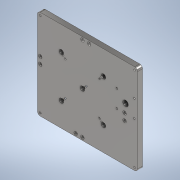
# Autodesk Inventor part: BasePlate
Saved by Autodesk Inventor 2022 (Build 260153070, 153G)
## iProperties
Company: UNC - Chapel Hill
Created: 2020-03-15
Part Number: BasePlate
Material: Stainless Steel
Document SubType Name: Modeling
Designer: elmar
Density: 8 g/cm^3
Appearance: Semi-Polished
BasePlateCornerRadius: 5.000 mm
BasePlateWidth: 160.000 mm
M3HoleDiameter: 3.200 mm
M3CounterSinkDiameter: 6.300 mm
MountHoleToSideDistance: 5.000 mm
Author: Eric L. Martin
Title: BasePlate
Autodesk Inventor part; units mm, degrees
ref_plane "YZ Plane" through (0, 0, 0) normal (1, 0, 0) x (0, 1, 0)
ref_plane "XZ Plane" through (0, 0, 0) normal (0, 1, 0) x (-1, 0, 0)
ref_plane "XY Plane" through (0, 0, 0) normal (0, 0, 1) x (1, 0, 0)
sketch "Sketch1" plane through (0, 0, 0) normal (0, 0, 1) x (1, 0, 0)
  line L0 (37.5, -37.5) -> (-37.5, -37.5)
  line L1 (-37.5, -37.5) -> (-37.5, 37.5)
  line L2 (-37.5, 37.5) -> (37.5, 37.5)
  line L3 (37.5, 37.5) -> (37.5, -37.5)
  line L4 (37.5, -37.5) -> (-37.5, 37.5) construction
  line L5 (-37.5, -37.5) -> (37.5, 37.5) construction
  line L6 (-75, 0) -> (0, 75)
  line L7 (0, 75) -> (75, 0)
  line L8 (75, 0) -> (0, -75)
  line L9 (0, -75) -> (-75, 0)
  line L10 (-115.5865, 0) -> (133.519, 0) projected
  circle A0 centre (37.5, 37.5) radius 37.5
  circle A1 centre (76.7825, 15.5482) radius 7.5
  circle A2 centre (37.5, -37.5) radius 38.5
  circle A3 centre (76.7825, 15.5482) radius 9.5
  line L11 (61.2825, 31.0482) -> (92.2825, 31.0482)
  line L12 (92.2825, 31.0482) -> (92.2825, 0.0482)
  line L13 (92.2825, 0.0482) -> (61.2825, 0.0482)
  line L14 (61.2825, 0.0482) -> (61.2825, 31.0482)
  line L15 (97.9325, 36.6982) -> (97.9325, -5.6018)
  line L16 (55.6325, -5.6018) -> (55.6325, 36.6982)
  line L17 (55.6325, 36.6982) -> (97.9325, 36.6982)
  line L18 (-80, 80) -> (97.9325, 80)
  line L19 (97.9325, 80) -> (97.9325, -80)
  line L20 (97.9325, -80) -> (-80, -80)
  line L21 (-80, -80) -> (-80, 80)
  circle A4 centre (76.7825, 15.5482) radius 11.5
  circle A5 centre (75, 0) radius 4.15
  circle A6 centre (61.2825, 0.0482) radius 4.15
  circle A7 centre (37.5, 37.5) radius 4
  circle A8 centre (0, 0) radius 4
  line L22 (3.9921, 0.2505) -> (0.2505, 3.9921)
  line L23 (37.2495, 33.5079) -> (33.5079, 37.2495)
  arc A9 (0.2505, 3.9921) -> (-1.3298, 3.7725) centre (-0.4566, 3.285) ccw
  arc A10 (3.7725, -1.3298) -> (3.9921, 0.2505) centre (3.285, -0.4566) ccw
  arc A11 (37.2495, 33.5079) -> (38.8298, 33.7275) centre (37.9566, 34.215) ccw
  arc A12 (33.7275, 38.8298) -> (33.5079, 37.2495) centre (34.215, 37.9566) ccw
  line L24 (36.7929, 34.6716) -> (34.6716, 32.5503)
  line L25 (34.6716, 32.5503) -> (32.5503, 34.6716)
  line L26 (32.5503, 34.6716) -> (34.6716, 36.7929)
  line L27 (34.6716, 36.7929) -> (36.7929, 34.6716)
  line L28 (36.7929, 34.6716) -> (32.5503, 34.6716) construction
  line L29 (34.6716, 32.5503) -> (34.6716, 36.7929) construction
  line L30 (2.8284, 0.7071) -> (4.9497, 2.8284)
  line L31 (4.9497, 2.8284) -> (2.8284, 4.9497)
  line L32 (2.8284, 4.9497) -> (0.7071, 2.8284)
  line L33 (0.7071, 2.8284) -> (2.8284, 0.7071)
  line L34 (2.8284, 0.7071) -> (2.8284, 4.9497) construction
  line L35 (4.9497, 2.8284) -> (0.7071, 2.8284) construction
  point P0 (-80, 0)
  point P1 (33.5, 37.5)
  point P2 (0, 37.5)
  point P3 (31.3564, 0.5067)
  point P4 (37.5, 1)
  point P5 (37.5, 33.5)
  point P6 (34.6716, 34.6716)
  point P7 (2.8284, 2.8284)
  point P8 (35.9386, 33.8173)
  point P9 (33.8173, 35.9386)
  point P10 (1.0607, 3.182)
  point P11 (3.182, 1.0607)
  point P12 (1.5614, 3.6827)
  point P13 (3.6827, 1.5614)
  dimension "d0" = 75
  dimension "d2" = 75
  dimension "d3" = 15
  dimension "d4" = 77
  dimension "d5" = 19
  dimension "StepperHoleSpacing" = 31
  dimension "StepperWidth" = 42.3
  dimension "StepperCountersinkDiameter" = 23
  dimension "d38" = 8.3
  dimension "d552" = 8.3
  dimension "d554" = 75
  dimension "d555" = 5
  dimension "MountHoleToSideDistance" = 5
  dimension "StepperToEdgeGap" = 0
  dimension "BasePlateWidth" = 160
  dimension "DistanceToCoveredHole" = 24.6421
  dimension "d764" = 8
  dimension "d777" = 3
  dimension "d793" = 1
  dimension "d794" = 3
  dimension "d795" = 3
  constraints: 70 end point, 18 point on circle, 13 centre point, 11 coincident, 10 parallel, 7 midpoint, 6 perpendicular, 6 tangent, 5 point on line, 4 equal length, 4 equal radius, 2 horizontal, 2 vertical, 25 other
  measures "d0" distance of L1.end L2.end
  measures "d2" diameter of A0
  measures "d3" diameter of A1
  measures "d4" diameter of A2
  measures "d5" diameter of A3
  measures "StepperHoleSpacing" distance of L11.start L11.end
  measures "StepperWidth" distance of L16.end L15.start
  measures "StepperCountersinkDiameter" diameter of A4
  measures "d38" diameter of A5
  measures "d552" diameter of A6
  measures "d554" distance of L7.end point (0, 0)
  measures "d555" distance from line of L18 L6.end
  measures "MountHoleToSideDistance" distance from line of L21 L6.start
  measures "StepperToEdgeGap" distance between parallel lines of L15 L19
  measures "BasePlateWidth" distance of L20.end L18.start
  measures "DistanceToCoveredHole" distance of L11.start L2.end
  measures "d764" diameter of A7
  measures "d777" distance between parallel lines of L7 L23
  measures "d793" radius of A9
  measures "d794" distance of L24.end L25.end
  measures "d795" distance of L25.end L26.end
extrude "Extrusion1" add sketch "Sketch1" along normal blind 9 contours L8 A2 L0 | L0 A2 L10 L3 | L3 L10 A2 L8 | L8 A2 | A2 L8 L9 L0 | L0 L1 L10 A8 A10 A2 | A0 A2 L3 | A0 A2 L10 | L10 A2 A0 | L3 A2 A0 | A2 L16 L10 A6 A5 L8 | L8 A5 L10 L15 L19 L20 L21 L9 A2 | L9 L10 L1 | L10 A10 A8 L30 L31 L32 A9 L1 L2 A0 A2 | A2 A0 L2 A12 A7 L26 L25 L24 A11 L3 | L3 A11 A7 L7 L16 A0 A2 | A2 A0 L16 L10 | L10 L16 A2 | A5 L10 L8 | L8 L10 A5 | L10 L6 L1 | L10 L21 L18 L19 L17 A0 L7 L6 | A10 A8 L10 | L10 A8 A10 | A11 A7 L3 | L3 A7 A11 | L16 A0 L14 A6 L10 | A0 L7 A7 A12 L2 | L2 L6 L7 A0 | L16 L7 L14 A0 | L10 A5 L13 L7 | L7 L13 A5 L10 | L10 A6 L13 A5 | A5 L13 L12 L11 A0 L17 L15 L10 | A8 L22 L32 L33 L30 L10 | L10 A8 | L22 L30 A8 | A7 L23 L24 L27 L26 L2 L3 | L3 L7 A7 | A7 L24 L23 | A6 L14 L13 L10 | L10 A6 | A12 A7 L2 | L2 A7 A12 | A0 L17 L16 L7 A7 | L14 L7 A0 | A0 L7 A5 L13 A6 L14 | L16 L17 A0 L11 L14 L7 | L13 A5 L7 | L7 A5 L13 | A5 A4 A0 L11 L12 L13 | A9 A8 | L30 L22 L32 A8 | A8 L32 L31 L30 | L30 L33 L32 L22 | L2 A7 L7 | L7 A7 | L24 L25 L26 A7 | A7 L26 L23 L24 | L23 L26 L27 L24 | A6 L13 L14 | L23 L26 A7 | A0 A4 A5 L7 | L7 L14 L11 A0 A4 | A4 A0 A3 | A8 L32 L22 | A4 A0 A3 | A3 A0 | A1 | A0 A3
fillet "Fillet1" radius 5 4 edges at (-80, 80, 4.5) (97.9325, 80, 4.5) (97.9325, -80, 4.5) (-80, -80, 4.5)
hole "Hole1" at (92.2825, 31.0482, 0) at (61.2825, 31.0482, 0) at (61.2825, 0.0482, 0) at (92.2825, 0.0482, 0) direction (0, 0, 1) diameter 3.2 depth 9 tip angle 118 countersink diameter 6.3 countersink angle 90 clearance for "Flat Head Machine Screw" size "M3" standard "Ansi Metric M Profile"
sketch "Sketch2" plane through (0, 0, 9) normal (0, 0, 1) x (1, 0, 0)
  circle A0 centre (76.7825, 15.5482) radius 11
  line L0 (75, 0) -> (75, -12)
  point P0 (0, 0)
  dimension "d660" = 22
  dimension "d773" = 12
  constraints: 2 coincident, 2 end point, 1 centre point, 1 vertical
  measures "d660" diameter of A0
  measures "d773" distance of L0.start L0.end
hole "Hole2" at (75, 0, 9) at (75, -12, 9) direction (0, 0, -1) diameter 3.2 depth 9 tip angle 118 countersink diameter 6.3 countersink angle 90 clearance for "Flat Head Machine Screw" size "M3" standard "Ansi Metric M Profile"
extrude "Extrusion7" cut sketch "Sketch1" along normal through all contours A7 L23 L24 L27 L26 L2 L3 | L3 L7 A7 | A7 L24 L23 | L2 A7 L7 | L7 A7 | L24 L25 L26 A7 | A7 L26 L23 L24 | L23 L26 L27 L24 | L23 L26 A7
pattern_circular "Circular Pattern1" count 4 over 360 about axis through (0, 0, -10) along (0, 0, 1) of "Extrusion7"
extrude "Extrusion8" cut sketch "Sketch1" along normal through all contours A8 L22 L32 L33 L30 L10 | L10 A8 | L22 L30 A8 | L30 L22 L32 A8 | A8 L32 L31 L30 | L30 L33 L32 L22 | A8 L32 L22
sketch "Sketch3" plane through (0, 0, 0) normal (0, 0, -1) x (-1, 0, 0)
  line L0 (-92.9325, 75) -> (75, 75)
  line L1 (75, 75) -> (75, -75)
  line L2 (75, -75) -> (-92.9325, -75)
  line L3 (-92.9325, -75) -> (-92.9325, 75)
  arc A0 (-92.9325, 80) -> (-97.9325, 75) centre (-92.9325, 75) ccw projected
  line L4 (117.6412, 0) -> (-138.5984, 0) projected
  arc A1 (80, 75) -> (75, 80) centre (75, 75) ccw projected
  line L5 (-101.9927, 46.55) -> (-59.6927, 46.55)
  line L6 (-59.6927, 46.55) -> (-59.6927, 4.25)
  line L7 (-59.6927, 4.25) -> (-101.9927, 4.25)
  line L8 (-101.9927, 4.25) -> (-101.9927, 46.55)
  point P0 (0, 0)
  point P1 (-92.9325, 0)
  point P2 (-80.8427, 25.4)
  point P3 (-80.8427, 25.4)
  dimension "d50" = 42.3
  constraints: 16 end point, 3 coincident, 2 horizontal, 2 parallel, 1 midpoint, 1 perpendicular, 1 point on line, 9 other
  measures "d50" distance of L7.end L5.start
hole "Hole4" at (92.9325, 75, 0) at (-75, 75, 0) at (-75, -75, 0) at (92.9325, -75, 0) direction (0, 0, 1) diameter 3.2 depth 9 tip angle 118 countersink diameter 6.3 countersink angle 90 clearance for "Flat Head Machine Screw" size "M3" standard "Ansi Metric M Profile"
hole "Hole7" at (76.7825, 15.5482, 0) direction (0, 0, 1) diameter 10 end through all
pattern_circular "Circular Pattern2" count 4 over 360 about axis through (0, 0, -10) along (0, 0, 1) of "Hole2"
ref_plane "Work Plane7" through (32.8221, 29.3997, 12.5355) normal (-0.5, -0.5, 0.7071068) x (-0.7071068, 0.7071068, 0)
ref_plane "Work Plane5" through (35.3221, 31.8997, 9) normal (-0.5, -0.5, 0.7071068) x (-0.7071068, 0.7071068, 0)
ref_plane "Work Plane6" through (19.8107, 17.6893, 0) normal (0.7071068, 0.7071068, 0) x (-0.7071068, 0.7071068, 0)
sketch "Sketch79" plane through (25.4285, 22.8162, 2.6523) normal (-0.5, -0.5, 0.7071068) x (-0.7071068, 0.7071068, 0)
  circle A0 centre (1.8472, -10.045) radius 1.5
  line L0 (3.3472, -7.6131) -> (0.3472, -7.6131) projected
  line L1 (0.3472, -13.977) -> (3.3472, -13.977) projected
  line L2 (1.8472, -13.977) -> (1.8472, -7.6131)
  point P0 (1.8472, 41.7426)
  point P1 (1.8472, -10.795)
  point P2 (1.8472, -10.795)
  dimension "d780" = 3
  dimension "d781" = 0.75
  constraints: 3 midpoint, 2 end point, 1 centre point, 1 coincident, 1 point on line
  measures "d780" diameter of A0
  measures "d781" distance of point (1.847, -10.795) A0.centre
hole "Hole9" at (29.5199, 29.5199, 10.2855) direction (0.5, 0.5, -0.7071068) diameter 2.459 end up to surface thread size "M3x0.5" class "6H" standard "ANSI Metric M Profile"
mirror "Mirror1" about plane through (19.8107, 17.6893, 0) normal (0.7071068, 0.7071068, 0) of "Hole9"
pattern_circular "Circular Pattern3" count 4 over 360 about axis through (0, 0, -10) along (0, 0, 1) of "Hole9"
equation "\"M3HoleDiameter\" = 3.2"
equation "\"M3CounterSinkDiameter\" = 6.3"
equation "\"d576\" = 55deg"
equation "\"Sketch57_Pitch\" = 1.25"
equation "\"d594\" = 55deg"
equation "\"Sketch59_Pitch\" = 1.25"
equation "\"d612\" = 55deg"
equation "\"Sketch61_Pitch\" = 1.25"
equation "\"d630\" = 55deg"
equation "\"Sketch63_Pitch\" = 1.25"
equation "\"d648\" = 55deg"
equation "\"Sketch65_Pitch\" = 1.25"
equation "\"d670\" = 55deg"
equation "\"Sketch67_Pitch\" = 1.25"
equation "\"d688\" = 55deg"
equation "\"Sketch69_Pitch\" = 1.25"
equation "\"d706\" = 55deg"
equation "\"Sketch71_Pitch\" = 1.25"
equation "\"d724\" = 55deg"
equation "\"Sketch73_Pitch\" = 1.25"
equation "\"d742\" = 55deg"
equation "\"Sketch75_Pitch\" = 1.25"
